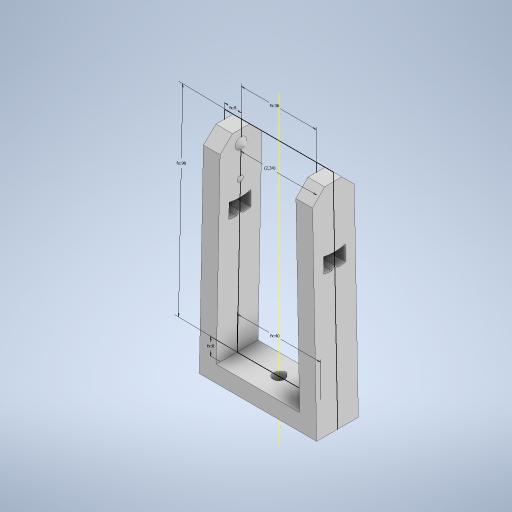
# Autodesk Inventor part: SolarFootAlt
Saved by Autodesk Inventor 2024.3 (Build 283343000, 343)
## iProperties
Created: 2025-02-03
Part Number: SolarFootAlt
Material: Generisch
Document SubType Name: Modeling
Designer: Maximilian Hock
Density: 1 g/cm^3
Appearance: Vorgabe
Author: Maximilian Hock
## iProperties of the stored document SolarFootAlt_3D-Druck.ipt
Created: 2025-02-06
Part Number: SolarFootAlt_3D-Druck
Material: Generisch
Document SubType Name: Modeling
Designer: maxho
Density: 1 g/cm^3
Appearance: Vorgabe
Author: maxho
Autodesk Inventor part; units mm, degrees
ref_plane "YZ Plane" through (0, 0, 0) normal (1, 0, 0) x (0, 1, 0)
ref_plane "XZ Plane" through (0, 0, 0) normal (0, 1, 0) x (-1, 0, 0)
ref_plane "XY Plane" through (0, 0, 0) normal (0, 0, 1) x (1, 0, 0)
sketch "Skizze1" plane through (0, 0, 0) normal (0, 1, 0) x (-1, 0, 0)
  line L0 (28.165, 0) -> (-28.165, 0)
  line L1 (-28.165, 0) -> (-26.0017, 105.9796)
  line L2 (-26.0017, 105.9796) -> (26.0017, 105.9796)
  line L3 (26.0017, 105.9796) -> (28.165, 0)
  line L4 (18, 105.9796) -> (-18, 105.9796)
  line L5 (-18, 105.9796) -> (-20, 8)
  line L6 (-20, 8) -> (20, 8)
  line L7 (20, 8) -> (18, 105.9796)
  line L8 (0, -20.9936) -> (0, 125.9617) projected
  point P0 (0, 0)
  point P1 (0, 8)
  point P2 (0, 0)
  dimension "d0" = 8
  dimension "d1" = 8
  dimension "d26" = 98
  dimension "d40" = 40
  dimension "d42" = 36
  dimension "d43" = 2.339
  constraints: 16 end point, 3 parallel, 2 coincident, 2 horizontal, 2 midpoint, 1 point on line, 1 vertical alignment, 1 other
  measures "d0" distance between parallel lines of L3 L7
  measures "d1" distance between parallel lines of L0 L6
  measures "d26" distance of L6.end L4.start
  measures "d40" distance of L5.end L6.end
  measures "d42" distance of L4.end L4.start
  measures "d43" angle of L5 L7
extrude "Extrusion1" add sketch "Skizze1" along normal mid plane 20 contours L0 L8 L6 L7 L2 L3 | L0 L1 L2 L5 L6 L8
sketch "Skizze2" plane through (0, 0, 0) normal (1, 0, 0) x (0, 1, 0)
  line L0 (10, 0) -> (-10, 0) projected
  line L1 (10, 105.9796) -> (10, 0) projected
  line L2 (-10, 105.9796) -> (10, 105.9796) projected
  line L3 (-10, 0) -> (-10, 105.9796) projected
  line L4 (-10, 105.9796) -> (-10, 0) projected
  arc A0 (0, 105.9796) -> (-10, 95.9796) centre (0, 95.9796) ccw
  arc A1 (10, 95.9796) -> (0, 105.9796) centre (0, 95.9796) ccw
  arc A2 (-5.2094, 66.4354) -> (5.2094, 66.4354) centre (0, 95.9796) ccw
  line L5 (0, 95.9796) -> (-5.2094, 66.4354)
  line L6 (5.2094, 66.4354) -> (0, 95.9796)
  arc A3 (-5.2094, 73.5773) -> (5.2094, 73.5773) centre (0, 95.9796) ccw
  line L7 (-1.4642, 66.0153) -> (0, 67.4796)
  line L8 (0, 67.4796) -> (1.4642, 66.0153)
  line L9 (-10, 95.9796) -> (0, 105.9796)
  line L10 (0, 105.9796) -> (10, 95.9796)
  line L11 (-4.1421, 101.8375) -> (4.1421, 101.8375)
  line L12 (-4.1421, 101.8375) -> (-10, 95.9796)
  line L13 (-5.2094, 66.4354) -> (-5.2094, 73.5773)
  line L14 (5.2094, 66.4354) -> (5.2094, 73.5773)
  point P0 (0, 0)
  point P1 (0, 0)
  point P2 (-3.9939, 73.329)
  point P3 (3.9939, 73.329)
  point P4 (0, 105.9796)
  point P5 (0, 65.9796)
  point P6 (0, 105.9796)
  point P7 (0, 105.9796)
  dimension "d12" = 30
  dimension "d27" = 7
  dimension "d28" = 1.5
  dimension "d29" = 20
  constraints: 21 end point, 13 point on circle, 6 point on line, 4 centre point, 4 coincident, 4 tangent, 3 midpoint, 2 equal length, 2 perpendicular, 2 vertical, 2 vertical alignment, 1 horizontal, 1 horizontal alignment
  measures "d12" radius of A2
  measures "d27" radial gap between concentric circles of A2 A3
  measures "d28" distance of point (0, 65.98) L7.end
  measures "d29" angle of L6 L5
extrude "Extrusion2" cut sketch "Skizze2" along normal through all both and the other way through all contours A1 L2 L1 | L10 A1 | L3 L2 A0 | A0 L9 | L10 L11 L9 | L5 A3 L6 A2 L8 L7 | L13 A3 L5 | A3 L14 L6
sketch "Skizze3" plane through (-20, -10, 8) normal (0.9997917, 0, -0.0204082) x (-0.0204082, 0, -0.9997917)
  circle A0 centre (-87.8346, 10) radius 2.7
  circle A1 centre (-72.8346, 10) radius 1.45
  point P0 (7.5902, 10)
  point P1 (-87.8346, 0)
  dimension "d18" = 5.4
  dimension "d19" = 2.9
  dimension "d20" = 15
  constraints: 2 centre point, 1 coincident, 1 horizontal alignment, 1 vertical alignment
  measures "d18" diameter of A0
  measures "d19" diameter of A1
  measures "d20" distance of point (-87.835, 10) A1.centre
extrude "Extrusion3" add sketch "Skizze3" along normal blind 10 draft -45 contours A0
extrude "Extrusion4" add sketch "Skizze3" along normal blind 5 draft -60 contours A1
mirror "Spiegeln1" about plane through (0, 0, 0) normal (1, 0, 0) of "Extrusion3", "Extrusion4"
sketch "Skizze4" plane through (-20, 10, 8) normal (0, 0, 1) x (1, 0, 0)
  line L0 (40, -20) -> (40, 0) projected
  line L1 (0, 0) -> (40, 0) projected
  line L2 (0, -20) -> (0, 0) projected
  line L3 (40, -20) -> (0, -20) projected
  point P0 (20, -10)
hole "Bohrung1" at (0, 0, 8) direction (0, 0, -1) diameter 5.5 end through all
sketch "Skizze5" plane through (-20, 10, 8) normal (0, 0, 1) x (1, 0, 0)
  circle A0 centre (20, -10) radius 2.75 projected
  line L0 (18.2989, -7.8393) -> (20, -6.5)
  line L1 (20, -6.5) -> (21.7011, -7.8393)
  dimension "d47" = 3.5
  constraints: 4 end point, 2 point on circle, 2 tangent, 1 vertical alignment
  measures "d47" distance of point (20, -10) L0.end
extrude "Extrusion5" cut sketch "Skizze5" against normal through all contours A0 L0 L1
sketch "Skizze6" plane through (28.165, 10, 0) normal (0, 0, -1) x (-1, 0, 0)
  line L0 (0, 0) -> (56.3299, 0) construction
  line L1 (56.3299, 0) -> (56.3299, -20) construction
  line L2 (56.3299, -20) -> (0, -20) construction
  line L3 (0, -20) -> (0, 0) construction
  spline S0 degree 2 poles (4.2488, -4.9266) (4.2488, -5.1847) (4.0588, -5.6073) (3.8744, -5.7548) knots 0 0 0 1 2 2 2
  spline S1 degree 2 poles (3.8744, -5.7548) (3.69, -5.9023) (3.188, -6.0611) (2.8278, -6.0611) knots 0 0 0 1 2 2 2
  spline S2 degree 2 poles (2.8278, -6.0611) (2.4194, -6.0611) (1.8351, -5.9249) (1.6507, -5.8399) knots 0 0 0 1 2 2 2
  line L4 (1.6507, -5.8399) -> (1.6507, -5.0797)
  line L5 (1.6507, -5.0797) -> (1.7358, -5.0797)
  spline S3 degree 2 poles (1.7358, -5.0797) (1.9287, -5.2017) (2.4477, -5.3832) (2.6633, -5.3832) knots 0 0 0 1 2 2 2
  spline S4 degree 2 poles (2.6633, -5.3832) (2.7909, -5.3832) (3.0887, -5.3378) (3.1908, -5.2641) knots 0 0 0 1 2 2 2
  spline S5 degree 2 poles (3.1908, -5.2641) (3.2703, -5.2045) (3.3667, -5.0315) (3.3667, -4.8755) knots 0 0 0 1 2 2 2
  spline S6 degree 2 poles (3.3667, -4.8755) (3.3667, -4.7195) (3.2306, -4.5522) (3.1171, -4.5125) knots 0 0 0 1 2 2 2
  spline S7 degree 2 poles (3.1171, -4.5125) (3.0036, -4.4728) (2.6888, -4.4642) (2.5669, -4.4642) knots 0 0 0 1 2 2 2
  line L6 (2.5669, -4.4642) -> (2.4165, -4.4642)
  line L7 (2.4165, -4.4642) -> (2.4165, -3.8488)
  line L8 (2.4165, -3.8488) -> (2.5555, -3.8488)
  spline S8 degree 2 poles (2.5555, -3.8488) (2.7143, -3.8488) (2.9838, -3.8204) (3.0774, -3.7779) knots 0 0 0 1 2 2 2
  spline S9 degree 2 poles (3.0774, -3.7779) (3.171, -3.7325) (3.2759, -3.5736) (3.2759, -3.4375) knots 0 0 0 1 2 2 2
  spline S10 degree 2 poles (3.2759, -3.4375) (3.2759, -3.3297) (3.1767, -3.1964) (3.1058, -3.1595) knots 0 0 0 1 2 2 2
  spline S11 degree 2 poles (3.1058, -3.1595) (3.0207, -3.117) (2.7938, -3.0886) (2.7143, -3.0886) knots 0 0 0 1 2 2 2
  spline S12 degree 2 poles (2.7143, -3.0886) (2.5867, -3.0886) (2.3173, -3.1482) (2.1925, -3.1964) knots 0 0 0 1 2 2 2
  spline S13 degree 2 poles (2.1925, -3.1964) (2.0932, -3.2333) (1.8776, -3.3524) (1.8266, -3.3836) knots 0 0 0 1 2 2 2
  line L9 (1.8266, -3.3836) -> (1.7528, -3.3836)
  line L10 (1.7528, -3.3836) -> (1.7528, -2.6348)
  spline S14 degree 2 poles (1.7528, -2.6348) (1.9344, -2.5583) (2.547, -2.4136) (2.8675, -2.4136) knots 0 0 0 1 2 2 2
  spline S15 degree 2 poles (2.8675, -2.4136) (3.1795, -2.4136) (3.639, -2.5214) (3.8006, -2.6263) knots 0 0 0 1 2 2 2
  spline S16 degree 2 poles (3.8006, -2.6263) (3.9793, -2.7369) (4.158, -3.0773) (4.158, -3.29) knots 0 0 0 1 2 2 2
  spline S17 degree 2 poles (4.158, -3.29) (4.158, -3.5907) (3.812, -4.0388) (3.5284, -4.104) knots 0 0 0 1 2 2 2
  line L11 (3.5284, -4.104) -> (3.5284, -4.1381)
  spline S18 degree 2 poles (3.5284, -4.1381) (3.6532, -4.1551) (3.8914, -4.2459) (4.0049, -4.348) knots 0 0 0 1 2 2 2
  spline S19 degree 2 poles (4.0049, -4.348) (4.1098, -4.4387) (4.2488, -4.728) (4.2488, -4.9266) knots 0 0 0 1 2 2 2
  line L12 (5.6414, -5.9873) -> (4.8104, -5.9873)
  line L13 (4.8104, -5.9873) -> (4.8104, -5.0627)
  line L14 (4.8104, -5.0627) -> (5.6414, -5.0627)
  line L15 (5.6414, -5.0627) -> (5.6414, -5.9873)
  line L16 (8.75, -5.9873) -> (6.4384, -5.9873)
  line L17 (6.4384, -5.9873) -> (6.4384, -5.3775)
  line L18 (6.4384, -5.3775) -> (7.1759, -5.3775)
  line L19 (7.1759, -5.3775) -> (7.1759, -3.5254)
  line L20 (7.1759, -3.5254) -> (6.4384, -3.5254)
  line L21 (6.4384, -3.5254) -> (6.4384, -2.9553)
  spline S20 degree 2 poles (6.4384, -2.9553) (6.6001, -2.9553) (6.9206, -2.9128) (7.017, -2.8674) knots 0 0 0 1 2 2 2
  spline S21 degree 2 poles (7.017, -2.8674) (7.1276, -2.8107) (7.2524, -2.6206) (7.2638, -2.4788) knots 0 0 0 1 2 2 2
  line L22 (7.2638, -2.4788) -> (8.0296, -2.4788)
  line L23 (8.0296, -2.4788) -> (8.0296, -5.3775)
  line L24 (8.0296, -5.3775) -> (8.75, -5.3775)
  line L25 (8.75, -5.3775) -> (8.75, -5.9873)
  line L26 (10.2107, -5.9873) -> (9.3797, -5.9873)
  line L27 (9.3797, -5.9873) -> (9.3797, -5.0627)
  line L28 (9.3797, -5.0627) -> (10.2107, -5.0627)
  line L29 (10.2107, -5.0627) -> (10.2107, -5.9873)
  line L30 (13.3193, -5.9873) -> (11.0077, -5.9873)
  line L31 (11.0077, -5.9873) -> (11.0077, -5.3775)
  line L32 (11.0077, -5.3775) -> (11.7451, -5.3775)
  line L33 (11.7451, -5.3775) -> (11.7451, -3.5254)
  line L34 (11.7451, -3.5254) -> (11.0077, -3.5254)
  line L35 (11.0077, -3.5254) -> (11.0077, -2.9553)
  spline S22 degree 2 poles (11.0077, -2.9553) (11.1694, -2.9553) (11.4899, -2.9128) (11.5863, -2.8674) knots 0 0 0 1 2 2 2
  spline S23 degree 2 poles (11.5863, -2.8674) (11.6969, -2.8107) (11.8217, -2.6206) (11.8331, -2.4788) knots 0 0 0 1 2 2 2
  line L36 (11.8331, -2.4788) -> (12.5989, -2.4788)
  line L37 (12.5989, -2.4788) -> (12.5989, -5.3775)
  line L38 (12.5989, -5.3775) -> (13.3193, -5.3775)
  line L39 (13.3193, -5.3775) -> (13.3193, -5.9873)
  spline S24 degree 2 poles (4.3282, -10.7771) (4.3282, -11.0012) (4.141, -11.3898) (3.9623, -11.5316) knots 0 0 0 1 2 2 2
  spline S25 degree 2 poles (3.9623, -11.5316) (3.7836, -11.6734) (3.2703, -11.8323) (2.9384, -11.8323) knots 0 0 0 1 2 2 2
  spline S26 degree 2 poles (2.9384, -11.8323) (2.5839, -11.8323) (2.0535, -11.6706) (1.8833, -11.5316) knots 0 0 0 1 2 2 2
  spline S27 degree 2 poles (1.8833, -11.5316) (1.716, -11.3926) (1.5571, -11.0154) (1.5571, -10.8055) knots 0 0 0 1 2 2 2
  spline S28 degree 2 poles (1.5571, -10.8055) (1.5571, -10.5049) (1.889, -10.1049) (2.2038, -9.9716) knots 0 0 0 1 2 2 2
  line L40 (2.2038, -9.9716) -> (2.2038, -9.9575)
  spline S29 degree 2 poles (2.2038, -9.9575) (1.8947, -9.8071) (1.6507, -9.3788) (1.6507, -9.1151) knots 0 0 0 1 2 2 2
  spline S30 degree 2 poles (1.6507, -9.1151) (1.6507, -8.9222) (1.8209, -8.5847) (1.9882, -8.4514) knots 0 0 0 1 2 2 2
  spline S31 degree 2 poles (1.9882, -8.4514) (2.1499, -8.3237) (2.6406, -8.1706) (2.9469, -8.1706) knots 0 0 0 1 2 2 2
  spline S32 degree 2 poles (2.9469, -8.1706) (3.2703, -8.1706) (3.7524, -8.3096) (3.9084, -8.423) knots 0 0 0 1 2 2 2
  spline S33 degree 2 poles (3.9084, -8.423) (4.0673, -8.5365) (4.2374, -8.8655) (4.2374, -9.0555) knots 0 0 0 1 2 2 2
  spline S34 degree 2 poles (4.2374, -9.0555) (4.2374, -9.3051) (3.9481, -9.705) (3.6503, -9.844) knots 0 0 0 1 2 2 2
  line L41 (3.6503, -9.844) -> (3.6503, -9.8553)
  spline S35 degree 2 poles (3.6503, -9.8553) (3.9992, -9.9972) (4.3282, -10.4566) (4.3282, -10.7771) knots 0 0 0 1 2 2 2
  spline S36 degree 2 poles (3.4603, -10.814) (3.4603, -10.641) (3.3128, -10.4595) (3.0746, -10.3432) knots 0 0 0 1 2 2 2
  spline S37 degree 2 poles (3.0746, -10.3432) (3.0065, -10.312) (2.7484, -10.2127) (2.6491, -10.1702) knots 0 0 0 1 2 2 2
  spline S38 degree 2 poles (2.6491, -10.1702) (2.5583, -10.2609) (2.4137, -10.5332) (2.4137, -10.6949) knots 0 0 0 1 2 2 2
  spline S39 degree 2 poles (2.4137, -10.6949) (2.4137, -10.9388) (2.7257, -11.231) (2.9781, -11.231) knots 0 0 0 1 2 2 2
  spline S40 degree 2 poles (2.9781, -11.231) (3.049, -11.231) (3.2249, -11.1856) (3.2929, -11.1402) knots 0 0 0 1 2 2 2
  spline S41 degree 2 poles (3.2929, -11.1402) (3.3695, -11.0863) (3.4603, -10.9388) (3.4603, -10.814) knots 0 0 0 1 2 2 2
  spline S42 degree 2 poles (3.3837, -9.1576) (3.3837, -8.9789) (3.1483, -8.7662) (2.9469, -8.7662) knots 0 0 0 1 2 2 2
  spline S43 degree 2 poles (2.9469, -8.7662) (2.7541, -8.7662) (2.5186, -8.9591) (2.5186, -9.1009) knots 0 0 0 1 2 2 2
  spline S44 degree 2 poles (2.5186, -9.1009) (2.5186, -9.2399) (2.6605, -9.4129) (2.8108, -9.4838) knots 0 0 0 1 2 2 2
  spline S45 degree 2 poles (2.8108, -9.4838) (2.876, -9.5178) (3.0575, -9.5887) (3.2079, -9.6455) knots 0 0 0 1 2 2 2
  spline S46 degree 2 poles (3.2079, -9.6455) (3.2986, -9.5263) (3.3837, -9.3023) (3.3837, -9.1576) knots 0 0 0 1 2 2 2
  line L42 (5.6414, -11.75) -> (4.8104, -11.75)
  line L43 (4.8104, -11.75) -> (4.8104, -10.8254)
  line L44 (4.8104, -10.8254) -> (5.6414, -10.8254)
  line L45 (5.6414, -10.8254) -> (5.6414, -11.75)
  spline S47 degree 2 poles (8.8606, -10) (8.8606, -10.4538) (8.716, -11.1345) (8.5543, -11.3643) knots 0 0 0 1 2 2 2
  spline S48 degree 2 poles (8.5543, -11.3643) (8.3955, -11.5912) (7.8821, -11.8237) (7.5134, -11.8237) knots 0 0 0 1 2 2 2
  spline S49 degree 2 poles (7.5134, -11.8237) (7.1418, -11.8237) (6.6313, -11.5912) (6.4696, -11.3586) knots 0 0 0 1 2 2 2
  spline S50 degree 2 poles (6.4696, -11.3586) (6.3079, -11.1288) (6.1633, -10.4538) (6.1633, -10) knots 0 0 0 1 2 2 2
  spline S51 degree 2 poles (6.1633, -10) (6.1633, -9.5348) (6.3079, -8.8768) (6.4724, -8.6386) knots 0 0 0 1 2 2 2
  spline S52 degree 2 poles (6.4724, -8.6386) (6.637, -8.406) (7.156, -8.1791) (7.5134, -8.1791) knots 0 0 0 1 2 2 2
  spline S53 degree 2 poles (7.5134, -8.1791) (7.8906, -8.1791) (8.3955, -8.4173) (8.5571, -8.6528) knots 0 0 0 1 2 2 2
  spline S54 degree 2 poles (8.5571, -8.6528) (8.716, -8.8825) (8.8606, -9.5604) (8.8606, -10) knots 0 0 0 1 2 2 2
  spline S55 degree 2 poles (7.9785, -10) (7.9785, -9.3505) (7.7658, -8.8258) (7.5134, -8.8258) knots 0 0 0 1 2 2 2
  spline S56 degree 2 poles (7.5134, -8.8258) (7.2609, -8.8258) (7.0454, -9.3505) (7.0454, -10.0028) knots 0 0 0 1 2 2 2
  spline S57 degree 2 poles (7.0454, -10.0028) (7.0454, -10.6438) (7.2609, -11.1771) (7.5134, -11.1771) knots 0 0 0 1 2 2 2
  spline S58 degree 2 poles (7.5134, -11.1771) (7.763, -11.1771) (7.9785, -10.6438) (7.9785, -10) knots 0 0 0 1 2 2 2
  line L46 (12.5109, -11.75) -> (12.5109, -10.4311)
  spline S59 degree 2 poles (12.5109, -10.4311) (12.5109, -10.2354) (12.4968, -9.9688) (12.4627, -9.8837) knots 0 0 0 1 2 2 2
  spline S60 degree 2 poles (12.4627, -9.8837) (12.4259, -9.7986) (12.2784, -9.722) (12.1451, -9.722) knots 0 0 0 1 2 2 2
  spline S61 degree 2 poles (12.1451, -9.722) (12.0515, -9.722) (11.8699, -9.8043) (11.7622, -9.8809) knots 0 0 0 1 2 2 2
  line L47 (11.7622, -9.8809) -> (11.7622, -11.75)
  line L48 (11.7622, -11.75) -> (10.934, -11.75)
  line L49 (10.934, -11.75) -> (10.934, -10.4311)
  spline S62 degree 2 poles (10.934, -10.4311) (10.934, -10.2382) (10.9169, -9.9688) (10.8829, -9.8837) knots 0 0 0 1 2 2 2
  spline S63 degree 2 poles (10.8829, -9.8837) (10.846, -9.7986) (10.6985, -9.722) (10.5652, -9.722) knots 0 0 0 1 2 2 2
  spline S64 degree 2 poles (10.5652, -9.722) (10.466, -9.722) (10.2703, -9.8156) (10.1795, -9.8809) knots 0 0 0 1 2 2 2
  line L50 (10.1795, -9.8809) -> (10.1795, -11.75)
  line L51 (10.1795, -11.75) -> (9.357, -11.75)
  line L52 (9.357, -11.75) -> (9.357, -9.1094)
  line L53 (9.357, -9.1094) -> (10.1795, -9.1094)
  line L54 (10.1795, -9.1094) -> (10.1795, -9.4015)
  spline S65 degree 2 poles (10.1795, -9.4015) (10.3809, -9.2314) (10.7411, -9.0385) (10.9652, -9.0385) knots 0 0 0 1 2 2 2
  spline S66 degree 2 poles (10.9652, -9.0385) (11.2062, -9.0385) (11.575, -9.2682) (11.6714, -9.498) knots 0 0 0 1 2 2 2
  spline S67 degree 2 poles (11.6714, -9.498) (11.9068, -9.2767) (12.3266, -9.0385) (12.5421, -9.0385) knots 0 0 0 1 2 2 2
  spline S68 degree 2 poles (12.5421, -9.0385) (12.7265, -9.0385) (13.0186, -9.1548) (13.1179, -9.2739) knots 0 0 0 1 2 2 2
  spline S69 degree 2 poles (13.1179, -9.2739) (13.2285, -9.4015) (13.3391, -9.7504) (13.3391, -10.0312) knots 0 0 0 1 2 2 2
  line L55 (13.3391, -10.0312) -> (13.3391, -11.75)
  line L56 (13.3391, -11.75) -> (12.5109, -11.75)
  line L57 (17.1001, -11.75) -> (17.1001, -10.4311)
  spline S70 degree 2 poles (17.1001, -10.4311) (17.1001, -10.2354) (17.0859, -9.9688) (17.0519, -9.8837) knots 0 0 0 1 2 2 2
  spline S71 degree 2 poles (17.0519, -9.8837) (17.015, -9.7986) (16.8675, -9.722) (16.7342, -9.722) knots 0 0 0 1 2 2 2
  spline S72 degree 2 poles (16.7342, -9.722) (16.6406, -9.722) (16.4591, -9.8043) (16.3513, -9.8809) knots 0 0 0 1 2 2 2
  line L58 (16.3513, -9.8809) -> (16.3513, -11.75)
  line L59 (16.3513, -11.75) -> (15.5231, -11.75)
  line L60 (15.5231, -11.75) -> (15.5231, -10.4311)
  spline S73 degree 2 poles (15.5231, -10.4311) (15.5231, -10.2382) (15.5061, -9.9688) (15.472, -9.8837) knots 0 0 0 1 2 2 2
  spline S74 degree 2 poles (15.472, -9.8837) (15.4352, -9.7986) (15.2877, -9.722) (15.1544, -9.722) knots 0 0 0 1 2 2 2
  spline S75 degree 2 poles (15.1544, -9.722) (15.0551, -9.722) (14.8594, -9.8156) (14.7686, -9.8809) knots 0 0 0 1 2 2 2
  line L61 (14.7686, -9.8809) -> (14.7686, -11.75)
  line L62 (14.7686, -11.75) -> (13.9461, -11.75)
  line L63 (13.9461, -11.75) -> (13.9461, -9.1094)
  line L64 (13.9461, -9.1094) -> (14.7686, -9.1094)
  line L65 (14.7686, -9.1094) -> (14.7686, -9.4015)
  spline S76 degree 2 poles (14.7686, -9.4015) (14.97, -9.2314) (15.3302, -9.0385) (15.5543, -9.0385) knots 0 0 0 1 2 2 2
  spline S77 degree 2 poles (15.5543, -9.0385) (15.7954, -9.0385) (16.1641, -9.2682) (16.2605, -9.498) knots 0 0 0 1 2 2 2
  spline S78 degree 2 poles (16.2605, -9.498) (16.4959, -9.2767) (16.9157, -9.0385) (17.1313, -9.0385) knots 0 0 0 1 2 2 2
  spline S79 degree 2 poles (17.1313, -9.0385) (17.3156, -9.0385) (17.6078, -9.1548) (17.707, -9.2739) knots 0 0 0 1 2 2 2
  spline S80 degree 2 poles (17.707, -9.2739) (17.8177, -9.4015) (17.9283, -9.7504) (17.9283, -10.0312) knots 0 0 0 1 2 2 2
  line L66 (17.9283, -10.0312) -> (17.9283, -11.75)
  line L67 (17.9283, -11.75) -> (17.1001, -11.75)
  line L68 (3.2249, -16.293) -> (1.6677, -16.293)
  line L69 (1.6677, -16.293) -> (1.6677, -15.6407)
  line L70 (1.6677, -15.6407) -> (3.2249, -15.6407)
  line L71 (3.2249, -15.6407) -> (3.2249, -16.293)
  line L72 (6.4554, -16.6958) -> (5.9818, -16.6958)
  line L73 (5.9818, -16.6958) -> (5.9818, -17.5212)
  line L74 (5.9818, -17.5212) -> (5.1337, -17.5212)
  line L75 (5.1337, -17.5212) -> (5.1337, -16.6958)
  line L76 (5.1337, -16.6958) -> (3.5908, -16.6958)
  line L77 (3.5908, -16.6958) -> (3.5908, -16.0435)
  line L78 (3.5908, -16.0435) -> (5.1053, -14.0127)
  line L79 (5.1053, -14.0127) -> (5.9818, -14.0127)
  line L80 (5.9818, -14.0127) -> (5.9818, -16.0661)
  line L81 (5.9818, -16.0661) -> (6.4554, -16.0661)
  line L82 (6.4554, -16.0661) -> (6.4554, -16.6958)
  line L83 (5.1337, -16.0661) -> (5.1337, -14.8749)
  line L84 (5.1337, -14.8749) -> (4.2459, -16.0661)
  line L85 (4.2459, -16.0661) -> (5.1337, -16.0661)
  line L86 (7.7176, -17.5127) -> (6.8865, -17.5127)
  line L87 (6.8865, -17.5127) -> (6.8865, -16.588)
  line L88 (6.8865, -16.588) -> (7.7176, -16.588)
  line L89 (7.7176, -16.588) -> (7.7176, -17.5127)
  spline S81 degree 2 poles (10.9368, -15.7627) (10.9368, -16.2165) (10.7921, -16.8972) (10.6305, -17.1269) knots 0 0 0 1 2 2 2
  spline S82 degree 2 poles (10.6305, -17.1269) (10.4716, -17.3538) (9.9583, -17.5864) (9.5895, -17.5864) knots 0 0 0 1 2 2 2
  spline S83 degree 2 poles (9.5895, -17.5864) (9.218, -17.5864) (8.7075, -17.3538) (8.5458, -17.1212) knots 0 0 0 1 2 2 2
  spline S84 degree 2 poles (8.5458, -17.1212) (8.3841, -16.8915) (8.2395, -16.2165) (8.2395, -15.7627) knots 0 0 0 1 2 2 2
  spline S85 degree 2 poles (8.2395, -15.7627) (8.2395, -15.2975) (8.3841, -14.6395) (8.5486, -14.4012) knots 0 0 0 1 2 2 2
  spline S86 degree 2 poles (8.5486, -14.4012) (8.7131, -14.1687) (9.2322, -13.9418) (9.5895, -13.9418) knots 0 0 0 1 2 2 2
  spline S87 degree 2 poles (9.5895, -13.9418) (9.9668, -13.9418) (10.4716, -14.18) (10.6333, -14.4154) knots 0 0 0 1 2 2 2
  spline S88 degree 2 poles (10.6333, -14.4154) (10.7921, -14.6452) (10.9368, -15.323) (10.9368, -15.7627) knots 0 0 0 1 2 2 2
  spline S89 degree 2 poles (10.0547, -15.7627) (10.0547, -15.1131) (9.842, -14.5884) (9.5895, -14.5884) knots 0 0 0 1 2 2 2
  spline S90 degree 2 poles (9.5895, -14.5884) (9.3371, -14.5884) (9.1216, -15.1131) (9.1216, -15.7655) knots 0 0 0 1 2 2 2
  spline S91 degree 2 poles (9.1216, -15.7655) (9.1216, -16.4065) (9.3371, -16.9397) (9.5895, -16.9397) knots 0 0 0 1 2 2 2
  spline S92 degree 2 poles (9.5895, -16.9397) (9.8391, -16.9397) (10.0547, -16.4065) (10.0547, -15.7627) knots 0 0 0 1 2 2 2
  line L90 (14.5871, -17.5127) -> (14.5871, -16.1938)
  spline S93 degree 2 poles (14.5871, -16.1938) (14.5871, -15.9981) (14.5729, -15.7315) (14.5389, -15.6464) knots 0 0 0 1 2 2 2
  spline S94 degree 2 poles (14.5389, -15.6464) (14.502, -15.5613) (14.3545, -15.4847) (14.2212, -15.4847) knots 0 0 0 1 2 2 2
  spline S95 degree 2 poles (14.2212, -15.4847) (14.1276, -15.4847) (13.9461, -15.567) (13.8383, -15.6435) knots 0 0 0 1 2 2 2
  line L91 (13.8383, -15.6435) -> (13.8383, -17.5127)
  line L92 (13.8383, -17.5127) -> (13.0101, -17.5127)
  line L93 (13.0101, -17.5127) -> (13.0101, -16.1938)
  spline S96 degree 2 poles (13.0101, -16.1938) (13.0101, -16.0009) (12.9931, -15.7315) (12.9591, -15.6464) knots 0 0 0 1 2 2 2
  spline S97 degree 2 poles (12.9591, -15.6464) (12.9222, -15.5613) (12.7747, -15.4847) (12.6414, -15.4847) knots 0 0 0 1 2 2 2
  spline S98 degree 2 poles (12.6414, -15.4847) (12.5421, -15.4847) (12.3464, -15.5783) (12.2557, -15.6435) knots 0 0 0 1 2 2 2
  line L94 (12.2557, -15.6435) -> (12.2557, -17.5127)
  line L95 (12.2557, -17.5127) -> (11.4331, -17.5127)
  line L96 (11.4331, -17.5127) -> (11.4331, -14.8721)
  line L97 (11.4331, -14.8721) -> (12.2557, -14.8721)
  line L98 (12.2557, -14.8721) -> (12.2557, -15.1642)
  spline S99 degree 2 poles (12.2557, -15.1642) (12.4571, -14.994) (12.8173, -14.8012) (13.0413, -14.8012) knots 0 0 0 1 2 2 2
  spline S100 degree 2 poles (13.0413, -14.8012) (13.2824, -14.8012) (13.6511, -15.0309) (13.7476, -15.2606) knots 0 0 0 1 2 2 2
  spline S101 degree 2 poles (13.7476, -15.2606) (13.983, -15.0394) (14.4028, -14.8012) (14.6183, -14.8012) knots 0 0 0 1 2 2 2
  spline S102 degree 2 poles (14.6183, -14.8012) (14.8027, -14.8012) (15.0948, -14.9174) (15.1941, -15.0366) knots 0 0 0 1 2 2 2
  spline S103 degree 2 poles (15.1941, -15.0366) (15.3047, -15.1642) (15.4153, -15.5131) (15.4153, -15.7939) knots 0 0 0 1 2 2 2
  line L99 (15.4153, -15.7939) -> (15.4153, -17.5127)
  line L100 (15.4153, -17.5127) -> (14.5871, -17.5127)
  line L101 (19.1763, -17.5127) -> (19.1763, -16.1938)
  spline S104 degree 2 poles (19.1763, -16.1938) (19.1763, -15.9981) (19.1621, -15.7315) (19.128, -15.6464) knots 0 0 0 1 2 2 2
  spline S105 degree 2 poles (19.128, -15.6464) (19.0912, -15.5613) (18.9437, -15.4847) (18.8104, -15.4847) knots 0 0 0 1 2 2 2
  spline S106 degree 2 poles (18.8104, -15.4847) (18.7168, -15.4847) (18.5353, -15.567) (18.4275, -15.6435) knots 0 0 0 1 2 2 2
  line L102 (18.4275, -15.6435) -> (18.4275, -17.5127)
  line L103 (18.4275, -17.5127) -> (17.5993, -17.5127)
  line L104 (17.5993, -17.5127) -> (17.5993, -16.1938)
  spline S107 degree 2 poles (17.5993, -16.1938) (17.5993, -16.0009) (17.5823, -15.7315) (17.5482, -15.6464) knots 0 0 0 1 2 2 2
  spline S108 degree 2 poles (17.5482, -15.6464) (17.5113, -15.5613) (17.3639, -15.4847) (17.2306, -15.4847) knots 0 0 0 1 2 2 2
  spline S109 degree 2 poles (17.2306, -15.4847) (17.1313, -15.4847) (16.9356, -15.5783) (16.8448, -15.6435) knots 0 0 0 1 2 2 2
  line L105 (16.8448, -15.6435) -> (16.8448, -17.5127)
  line L106 (16.8448, -17.5127) -> (16.0223, -17.5127)
  line L107 (16.0223, -17.5127) -> (16.0223, -14.8721)
  line L108 (16.0223, -14.8721) -> (16.8448, -14.8721)
  line L109 (16.8448, -14.8721) -> (16.8448, -15.1642)
  spline S110 degree 2 poles (16.8448, -15.1642) (17.0462, -14.994) (17.4064, -14.8012) (17.6305, -14.8012) knots 0 0 0 1 2 2 2
  spline S111 degree 2 poles (17.6305, -14.8012) (17.8716, -14.8012) (18.2403, -15.0309) (18.3367, -15.2606) knots 0 0 0 1 2 2 2
  spline S112 degree 2 poles (18.3367, -15.2606) (18.5721, -15.0394) (18.9919, -14.8012) (19.2075, -14.8012) knots 0 0 0 1 2 2 2
  spline S113 degree 2 poles (19.2075, -14.8012) (19.3918, -14.8012) (19.684, -14.9174) (19.7832, -15.0366) knots 0 0 0 1 2 2 2
  spline S114 degree 2 poles (19.7832, -15.0366) (19.8938, -15.1642) (20.0045, -15.5131) (20.0045, -15.7939) knots 0 0 0 1 2 2 2
  line L110 (20.0045, -15.7939) -> (20.0045, -17.5127)
  line L111 (20.0045, -17.5127) -> (19.1763, -17.5127)
  point P0 (28.165, -10)
  dimension "FootThickness" = 8
  dimension "SolarScalePreTension" = 4
  constraints: 2 coincident, 2 other
emboss "Prägen1" sketch "Skizze6" operation cut depth 0.5 direction (0, 0, 1)
equation "\"d0\" = FootThickness"
equation "\"d1\" = d0"
equation "\"d26\" = FootHeight"
equation "\"d40\" = SolarScaleThickness"
equation "\"d42\" = d40 - SolarScalePreTension"
equation "\"d2\" = 2 * SolarScaleAxleOffset"
equation "\"d12\" = SolarScaleRadius"
equation "\"d18\" = SolarScaleAxleDiameter + 2 * Clearance"
equation "\"d19\" = SolarScaleRatchetHoleDiameter + 2 * Clearance"
equation "\"FootHeight\" = 98"
equation "\"SolarScaleThickness\" = 40"
equation "\"SolarScaleAxleOffset\" = 10"
equation "\"SolarScaleRadius\" = 30"
equation "\"SolarScaleAxleDiameter\" = 5"
equation "\"Clearance\" = 0.2"
equation "\"SolarScaleRatchetHoleDiameter\" = 2.5"
